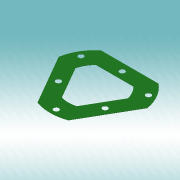
# Autodesk Inventor part: スプリングフランジ
Saved by Autodesk Inventor 2015 (Build 190159000, 159)
## iProperties
Created: 2016-02-18
Part Number: スプリングフランジ
Material: 一般
Document SubType Name: Modeling
Designer: buzztaka
Density: 1 g/cm^3
Appearance: 滑らか - 濃い深緑
Author: buzztaka
Autodesk Inventor part; units mm, degrees
ref_plane "YZ Plane" through (0, 0, 0) normal (1, 0, 0) x (0, 1, 0)
ref_plane "XZ Plane" through (0, 0, 0) normal (0, 1, 0) x (-1, 0, 0)
ref_plane "XY Plane" through (0, 0, 0) normal (0, 0, 1) x (1, 0, 0)
sketch "スケッチ1" plane through (0, 0, 0) normal (0, 0, 1) x (1, 0, 0)
  arc A0 (29.5493, 5.1808) -> (19.2614, 23) centre (0, 0) ccw
  arc A1 (-19.2614, 23) -> (-29.5493, 5.1808) centre (0, 0) ccw
  arc A2 (-10.2879, -28.1808) -> (10.2879, -28.1808) centre (0, 0) ccw
  line L0 (29.5493, 5.1808) -> (10.2879, -28.1808)
  line L1 (0, 23) -> (19.2614, 23)
  line L2 (19.9186, -11.5) -> (29.5493, 5.1808)
  line L3 (-19.9186, -11.5) -> (-29.5493, 5.1808)
  line L4 (19.2614, 23) -> (-19.2614, 23)
  line L5 (-29.5493, 5.1808) -> (-10.2879, -28.1808)
  arc A3 (17.4833, 4.2819) -> (12.4499, 13) centre (0, 0) ccw
  arc A4 (-12.4499, 13) -> (-17.4833, 4.2819) centre (0, 0) ccw
  arc A5 (-5.0334, -17.2819) -> (5.0334, -17.2819) centre (0, 0) ccw
  line L6 (0, 13) -> (12.4499, 13)
  line L7 (17.4833, 4.2819) -> (5.0334, -17.2819)
  line L8 (-11.2583, -6.5) -> (-17.4833, 4.2819)
  line L9 (0, 13) -> (-12.4499, 13)
  line L10 (-17.4833, 4.2819) -> (-5.0334, -17.2819)
  point P0 (11.2583, -6.5)
  dimension "d10" = 360
  dimension "d6" = 23
  constraints: 22 end point, 12 point on circle, 6 centre point, 6 coincident, 2 horizontal, 8 other
  measures "d6" distance of A0.centre L1.start
extrude "押し出し1" add sketch "スケッチ1" along normal blind 0.1
sketch "スケッチ2" plane through (0, 0, 0.1) normal (0, 0, 1) x (1, 0, 0)
  point P0 (0, 0)
  point P1 (0, 18)
  point P2 (0, 0)
  point P3 (-15.5885, -9)
  point P4 (0, 0)
  point P5 (15.5885, -9)
  point P6 (0, -26)
  point P7 (22.5167, 13)
  point P8 (-22.5167, 13)
  dimension "d15" = 18
  dimension "d18" = 360
  dimension "d20" = 26
  dimension "d23" = 360
  constraints: 2 coincident, 9 other
  measures "d15" distance of point (0, 0) point (0, 18)
  measures "d20" distance of point (0, -26) point (0, 0)
hole "穴1" at (0, 18, 0.1) at (-15.5885, -9, 0.1) at (15.5885, -9, 0.1) at (0, -26, 0.1) at (22.5167, 13, 0.1) at (-22.5167, 13, 0.1) direction (0, 0, -1) diameter 3.5 end through all
